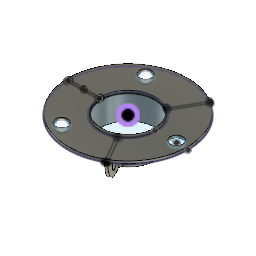
MFJ-1910-yoke (Autodesk Fusion 360 design; units mm, degrees)
Autodesk Fusion 360 part; units mm, degrees
sketch "Sketch1" plane through (0, 0, 0) normal (0, 0, 1) x (1, 0, 0)
  circle A0 centre (0, 0) radius 22.225
  circle A1 centre (0, 0) radius 23.225
  circle A2 centre (0, 0) radius 48.225
  circle A3 centre (0, 0) radius 21.725
  dimension "d4" = 44.45
  dimension "d6" = 46.45
  dimension "d8" = 96.45
  dimension "d11" = 43.45
  constraint coincident A0.centre A1.centre
  constraint concentric A0 A1
  constraint concentric A1 A2
  constraint concentric A0 A3
  measures "d4" diameter of A0
  measures "d6" diameter of A1
  measures "d8" diameter of A2
  measures "d11" diameter of A3
extrude "Extrude1" add sketch "Sketch1" along normal blind 2 contours A0 | A1 | A2 picked at (-3.813557, 21.670312) picked at (22.805199, -1.153836) picked at (39.625654, -3.54969) makes body 1
extrude "Extrude2" add sketch "Sketch1" against normal blind 20 contours A1 picked at (22.805199, -1.153836) bodies 1
sketch "Sketch2" plane through (0, 0, 0) normal (0, 0, 1) x (1, 0, 0)
  line L0 (48.224952, 0.067907) -> (21.724894, 0.067907) construction
  circle A0 centre (0, 0) radius 21.725 construction
  circle A1 centre (0, 0) radius 48.225 construction
  circle A2 centre (39.224952, 0.067907) radius 5
  circle A3 centre (-19.671285, 33.935852) radius 5
  circle A4 centre (-19.553667, -34.003758) radius 5
  dimension "d16" = 10
  dimension "d17" = 9
  dimension "d19" = 360
  constraint horizontal L0
  measures "d16" diameter of A2
extrude "Extrude3" cut sketch "Sketch2" along normal up to surface (2 mm away) contours A2 | A3 | A4 picked at (38.707057, 1.387482) picked at (-21.1729, 33.212712) picked at (-21.055282, -34.726898) bodies 1
sketch "Sketch3" plane through (0, 0, 0) normal (0, 0, 1) x (1, 0, 0)
  line L0 (-48.225, 0.000006) -> (-23.225, 0.000006) construction
  circle A0 centre (0, 0) radius 48.225
  circle A1 centre (0, 0) radius 23.225
  line L1 (-23.203461, 1) -> (-48.214631, 1)
  line L2 (-48.214631, 1) -> (-48.214631, -1)
  line L3 (-48.214631, -1) -> (-23.203461, -1)
  line L4 (-23.203461, -1) -> (-23.203461, 1)
  line L5 (-23.203461, 1) -> (-48.214631, -1) construction
  line L6 (-48.214631, 1) -> (-23.203461, -1) construction
  line L7 (10.735705, -20.594787) -> (23.24129, -42.255095)
  line L8 (24.973341, -41.255095) -> (12.467756, -19.594787)
  line L9 (12.467756, 19.594787) -> (24.973341, 41.255095)
  line L10 (23.24129, 42.255095) -> (10.735705, 20.594787)
  point P0 (-35.709046, 0)
  dimension "d22" = 2
  dimension "d24" = 360
  constraint horizontal L0
  constraint horizontal L1
  constraint perpendicular L1 L2
  constraint parallel L1 L3
extrude "Extrude5" add sketch "Sketch3" against normal up to surface (20 mm away) separate body contours A0 A1 L9 L10 picked at (15.681946, 27.384163) makes body 2
fillet "Fillet2" radius 20 1 edges at (24.1125, 41.764075, -20) on bodies 2
sketch "Sketch4" plane through (-0.866025, 0.5, 0) normal (-0.8660254, 0.5, 0) x (-0.5, -0.8660254, 0)
  spline S0 degree 3 poles (-28.20728, -20) (-29.442224, -20) (-30.790956, -19.87823) (-33.4324, -19.353007) (-34.725112, -18.94955) (-37.006562, -18.004714) (-38.205529, -17.376386) (-40.443965, -15.880989) (-41.483433, -15.013918) (-43.229085, -13.2685) (-44.096131, -12.229388) (-45.591535, -9.991658) (-46.219891, -8.79304) (-47.164499, -6.512793) (-47.5678, -5.221101) (-48.092866, -2.581711) (-48.214631, -1.234012) (-48.214631, 0) knots -2.96250966 -2.96250966 -2.96250966 -2.96250966 -2.59202639 -2.59202639 -2.22154311 -2.22154311 -1.85121924 -1.85121924 -1.48089538 -1.48089538 -1.11065128 -1.11065128 -0.74040719 -0.74040719 -0.3702036 -0.3702036 0 0 0 0
  line L0 (-28.20728, -20) -> (-23.203461, -20)
  line L1 (-23.203461, -20) -> (-23.203461, 0)
  line L2 (-23.203461, 0) -> (-48.214631, 0)
  line L3 (-23.203461, 0) -> (-39.626532, -16.42307) construction
  line L4 (-23.203461, 0) -> (0.42541, 0) construction
  circle A0 centre (-33.262571, -10.059109) radius 5
  dimension "d33" = 135
  dimension "d34" = 10
  dimension "d35" = 9
  constraint horizontal L4
  measures "d33" angle of L3 L4
  measures "d34" diameter of A0
extrude "Extrude6" cut sketch "Sketch4" against normal up to surface (2 mm away) contours A0 picked at (-33.32195, -11.435585) bodies 2
pattern_circular "C-Pattern1" count 3 over 360 about axis through (0, 0, 1.75) along (0, 0, 1) of bodies 2 makes body 3 at (-35.018104, 1, -1.69103) makes body 4 at (16.643027, -30.826568, -1.69103)
combine "Combine2" operation add target body 1 tool bodies 2 3 4
fillet "Fillet3" radius 2 1 edges at (10.735705, 20.594787, -10) on bodies 1
fillet "Fillet3" radius 2 11 edges at (16.988498, 31.424941, 0) (-23.203461, 1, -10) (-35.709046, 1, 0) (12.467756, 19.594787, -10) (18.720548, 30.424941, 0) (12.467756, -19.594787, -10) (18.720548, -30.424941, 0) (16.988498, -31.424941, 0) (10.735705, -20.594787, -10) (-23.203461, -1, -10) (-35.709046, -1, 0) on bodies 1
equation "tube_diameter = 1.75 in"
equation "eyelet_diameter = 10 mm"
equation "tube_overhang = 0.5 mm"
equation "d4 = tube_diameter"
equation "outer_diameter = tube_diameter + edge_thickness"
equation "d6 = outer_diameter"
equation "shelf_diameter = outer_diameter + 50 mm"
equation "d8 = shelf_diameter"
equation "edge_thickness = 2 mm"
equation "sleeve_height = 20 mm"
equation "d11 = tube_diameter - tube_overhang * 2"
equation "d12 = edge_thickness"
equation "d14 = -sleeve_height"
equation "d16 = eyelet_diameter"
equation "d17 = eyelet_diameter / 2 + edge_thickness * 2"
equation "d22 = edge_thickness"
equation "d32 = sleeve_height"
equation "d34 = eyelet_diameter"
equation "d35 = ( eyelet_diameter / 2 ) + edge_thickness * 2"
equation "d41 = edge_thickness"
equation "d43 = edge_thickness"
